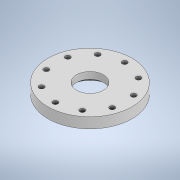
# Autodesk Inventor part: Крышка сальников
Saved by Autodesk Inventor 2021 (Build 250183000, 183)
## iProperties
Created: 2020-11-05
Part Number: Крышка сальников
Material: Типовые
Document SubType Name: Modeling
Designer: Тимоха
Density: 1 g/cm^3
Appearance: По умолчанию
Author: Тимоха
Autodesk Inventor part; units mm, degrees
ref_plane "YZ Plane" through (0, 0, 0) normal (1, 0, 0) x (0, 1, 0)
ref_plane "XZ Plane" through (0, 0, 0) normal (0, 1, 0) x (-1, 0, 0)
ref_plane "XY Plane" through (0, 0, 0) normal (0, 0, 1) x (1, 0, 0)
sketch "Эскиз1" plane through (0, 0, 0) normal (0, 0, 1) x (1, 0, 0)
  line L0 (0, 0) -> (0, 18)
  line L1 (0, 18) -> (100, 18)
  line L2 (100, 18) -> (100, -7)
  line L3 (100, -7) -> (70, -7)
  line L4 (70, -7) -> (70, -13)
  line L5 (70, -13) -> (50, -13)
  line L6 (50, -13) -> (50, 2)
  line L7 (50, 2) -> (32, 2)
  line L8 (32, 2) -> (32, 18)
  dimension "d7" = 18
  dimension "d8" = 100
  dimension "d9" = 25
  dimension "d10" = 30
  dimension "d11" = 20
  dimension "d12" = 15
  dimension "d13" = 18
  dimension "d26" = 16
  constraints: 18 end point, 6 perpendicular, 2 vertical, 1 horizontal, 1 point on line
  measures "d7" distance of L0.start L0.end
  measures "d8" distance of L0.end L1.end
  measures "d9" distance of L1.end L2.end
  measures "d10" distance of L2.end L3.end
  measures "d11" distance of L4.end L5.end
  measures "d12" distance of L5.end L6.end
  measures "d13" distance of L6.end L7.end
  measures "d26" distance of L7.end L8.end
revolve "Вращение1" add sketch "Эскиз1" angle 360 about axis through (0, 0, 0) along (0, 1, 0)
sketch "Эскиз2" plane through (0, 18, 0) normal (0, 1, 0) x (1, 0, 0)
  circle A0 centre (0, 0) radius 100 projected
  circle A1 centre (0, 0) radius 100 projected
  line L0 (0, 100) -> (0, 82.5)
  dimension "d15" = 17.5
  constraints: 2 end point, 1 vertical, 1 vertical alignment, 1 other
  measures "d15" distance of L0.start L0.end
hole "Отверстие1" at (0, 18, -82.5) direction (0, -1, 0) diameter 12 end through all
pattern_circular "Круговой массив1" count 10 over 360 about axis through (0, 10, 0) along (0, -1, 0) of "Отверстие1"
